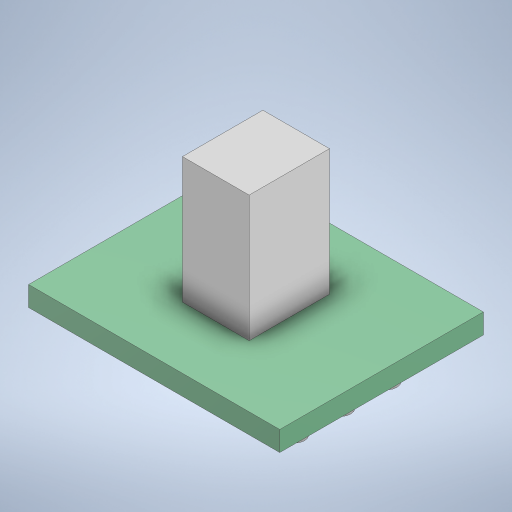
# Autodesk Inventor part: IF Remote reader
Saved by Autodesk Inventor 2023 (Build 270158000, 158)
## iProperties
Created: 2023-10-14
Part Number: IF Remote reader
Material: Generic
Document SubType Name: Modeling
Designer: Gage
Density: 1 g/cm^3
Appearance: Default
Author: Gage
Autodesk Inventor part; units mm, degrees
ref_plane "YZ Plane" through (0, 0, 0) normal (1, 0, 0) x (0, 1, 0)
ref_plane "XZ Plane" through (0, 0, 0) normal (0, 1, 0) x (-1, 0, 0)
ref_plane "XY Plane" through (0, 0, 0) normal (0, 0, 1) x (1, 0, 0)
sketch "Sketch1" plane through (0, 0, 0) normal (0, 1, 0) x (-1, 0, 0)
  line L0 (9.6647, -7.8359) -> (-9.6647, -7.8359)
  line L1 (-9.6647, -7.8359) -> (-9.6647, 7.8359)
  line L2 (-9.6647, 7.8359) -> (9.6647, 7.8359)
  line L3 (9.6647, 7.8359) -> (9.6647, -7.8359)
  point P0 (0, 0)
  point P1 (-9.6647, 0)
  point P2 (0, -7.8359)
  dimension "d0" = 19.3294
  dimension "d1" = 15.6718
  constraints: 8 end point, 2 midpoint, 2 parallel, 1 horizontal, 1 horizontal alignment, 1 perpendicular, 1 vertical alignment
  measures "d0" distance of L1.end L2.end
  measures "d1" distance of L0.end L1.end
extrude "Extrusion1" add sketch "Sketch1" along normal blind 1.5367
sketch "Sketch2" plane through (0, 1.5367, 0) normal (0, 1, 0) x (1, 0, 0)
  line L0 (-2.5654, -3.0925) -> (2.5654, -3.0925)
  line L1 (2.5654, -3.0925) -> (2.5654, 3.0925)
  line L2 (2.5654, 3.0925) -> (-2.5654, 3.0925)
  line L3 (-2.5654, 3.0925) -> (-2.5654, -3.0925)
  point P0 (0, 0)
  point P1 (-2.5654, 0)
  point P2 (0, 3.0925)
  dimension "d4" = 5.1308
  dimension "d5" = 6.1849
  constraints: 8 end point, 2 midpoint, 2 parallel, 1 horizontal, 1 horizontal alignment, 1 perpendicular, 1 vertical alignment
  measures "d4" distance of L2.end L1.end
  measures "d5" distance of L1.end L0.end
extrude "Extrusion2" add sketch "Sketch2" along normal blind 9.7028
sketch "Sketch3" plane through (0, 0, 0) normal (0, -1, 0) x (1, 0, 0)
  circle A0 centre (51.2064, 25.6032) radius 0.8001
  circle A1 centre (6.4897, 3.556) radius 0.8001
  circle A2 centre (6.4897, 0) radius 0.8001
  circle A3 centre (6.4897, -3.556) radius 0.8001
  line L0 (9.6647, 7.8359) -> (9.6647, -7.8359) projected
  point P0 (0, 0)
  dimension "d8" = 1.6002
  dimension "d9" = 1.6002
  dimension "d10" = 1.6002
  dimension "d11" = 7.112
  dimension "d12" = 3.556
  dimension "d13" = 3.175
  dimension "d14" = 3.175
  constraints: 4 centre point, 1 horizontal alignment
  measures "d8" diameter of A0
  measures "d9" diameter of A1
  measures "d10" diameter of A2
  measures "d11" distance of A3.centre A1.centre
  measures "d12" distance of A3.centre A2.centre
  measures "d13" distance from line of L0 A1.centre
  measures "d14" distance from line of L0 A2.centre
extrude "Extrusion3" add sketch "Sketch3" along normal blind 2.54 contours A1 | A2 | A3
body "Solid1"
